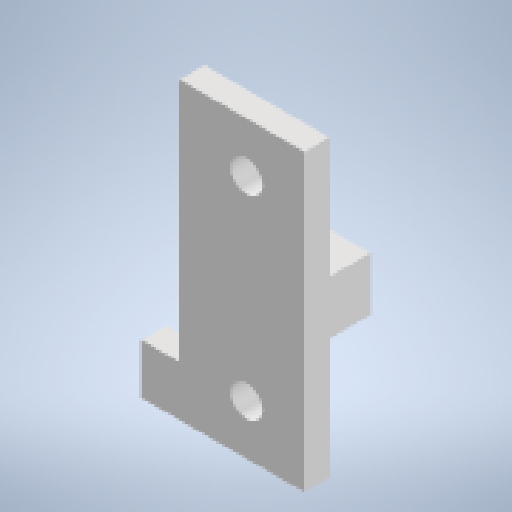
# Autodesk Inventor part: крышка
Saved by Autodesk Inventor 2024.2 (Build 282272000, 272)
## iProperties
Created: 2026-02-19
Part Number: крышка
Material: Типовые
Document SubType Name: Modeling
Designer: katya_notebook
Density: 1 g/cm^3
Appearance: По умолчанию
Author: katya_notebook
Autodesk Inventor part; units mm, degrees
ref_plane "YZ Plane" through (0, 0, 0) normal (1, 0, 0) x (0, 1, 0)
ref_plane "XZ Plane" through (0, 0, 0) normal (0, 1, 0) x (-1, 0, 0)
sketch "Эскиз1" plane through (0, 0, 0) normal (0, 0, 1) x (1, 0, 0)
  circle A0 centre (0.3813, 7.7585) radius 1.25 projected
  line L0 (-4.9754, 3.7665) -> (-4.9754, 11.75) projected
  line L1 (5, 3.7665) -> (-4.9754, 3.7665) projected
  line L2 (5, 11.75) -> (5, 3.7665) projected
  line L3 (-4.9754, 11.75) -> (5, 11.75) projected
  arc A1 (1.6313, -7.75) -> (-0.8686, -7.75) centre (0.3813, -7.762) ccw projected
  line L4 (-0.8686, -7.75) -> (1.6313, -7.75) projected
  line L5 (5, -11.75) -> (-8, -11.75) projected
  line L6 (5, -3.7735) -> (5, -11.75) projected
  line L7 (-5, -3.7735) -> (5, -3.7735) projected
  line L8 (-5, -7.75) -> (-5, -3.7735) projected
  line L9 (-8, -7.75) -> (-5, -7.75) projected
  line L10 (-8, -11.75) -> (-8, -7.75) projected
  line L11 (3.0114, -0.7535) -> (3.0052, -0.7535) projected
  line L12 (3.0114, -0.7535) -> (3.0114, -0.7535) projected
  arc A2 (3.5595, -1.3518) -> (3.0114, -0.7535) centre (3.0062, -1.3085) ccw projected
  arc A3 (3.5595, -1.3518) -> (3.709, -1.5135) centre (3.709, -1.3635) ccw projected
  line L13 (4.3002, -1.5135) -> (3.709, -1.5135) projected
  arc A4 (4.3002, -1.5135) -> (4.4502, -1.3635) centre (4.3002, -1.3635) ccw projected
  line L14 (4.4502, -1.2761) -> (4.4502, -1.3635) projected
  line L15 (4.4521, -1.2761) -> (4.4502, -1.2761) projected
  arc A5 (5, -0.7535) -> (4.4521, -1.2761) centre (5.0062, -1.3085) ccw projected
  line L16 (5, 0.7465) -> (5, -0.7535) projected
  arc A6 (4.4521, 1.2691) -> (5, 0.7465) centre (5.0062, 1.3015) ccw projected
  line L17 (4.4502, 1.2691) -> (4.4521, 1.2691) projected
  line L18 (4.4502, 1.3565) -> (4.4502, 1.2691) projected
  arc A7 (4.4502, 1.3565) -> (4.3002, 1.5065) centre (4.3002, 1.3565) ccw projected
  line L19 (3.709, 1.5065) -> (4.3002, 1.5065) projected
  arc A8 (3.709, 1.5065) -> (3.5595, 1.3448) centre (3.709, 1.3565) ccw projected
  arc A9 (3.0114, 0.7465) -> (3.5595, 1.3448) centre (3.0062, 1.3015) ccw projected
  line L20 (3.0114, 0.7465) -> (3.0114, 0.7465) projected
  line L21 (3.0052, 0.7465) -> (3.0114, 0.7465) projected
  line L22 (3.0052, 0.7465) -> (3.0052, 0.7465) projected
  arc A10 (2.4583, 1.2691) -> (3.0052, 0.7465) centre (3.0123, 1.3015) ccw projected
  line L23 (2.4564, 1.2691) -> (2.4583, 1.2691) projected
  line L24 (2.4564, 1.3565) -> (2.4564, 1.2691) projected
  arc A11 (2.4564, 1.3565) -> (2.3064, 1.5065) centre (2.3064, 1.3565) ccw projected
  line L25 (1.7152, 1.5065) -> (2.3064, 1.5065) projected
  arc A12 (1.7152, 1.5065) -> (1.5656, 1.3448) centre (1.7152, 1.3565) ccw projected
  arc A13 (1.0175, 0.7465) -> (1.5656, 1.3448) centre (1.0123, 1.3015) ccw projected
  line L26 (1.0175, 0.7465) -> (1.0175, 0.7465) projected
  line L27 (1.0114, 0.7465) -> (1.0175, 0.7465) projected
  line L28 (1.0114, 0.7465) -> (1.0114, 0.7465) projected
  arc A14 (0.4644, 1.2691) -> (1.0114, 0.7465) centre (1.0185, 1.3015) ccw projected
  line L29 (0.4625, 1.2691) -> (0.4644, 1.2691) projected
  line L30 (0.4625, 1.3565) -> (0.4625, 1.2691) projected
  arc A15 (0.4625, 1.3565) -> (0.3125, 1.5065) centre (0.3125, 1.3565) ccw projected
  line L31 (-0.2787, 1.5065) -> (0.3125, 1.5065) projected
  arc A16 (-0.2787, 1.5065) -> (-0.4282, 1.3448) centre (-0.2787, 1.3565) ccw projected
  arc A17 (-0.9763, 0.7465) -> (-0.4282, 1.3448) centre (-0.9815, 1.3015) ccw projected
  line L32 (-0.9763, 0.7465) -> (-0.9763, 0.7465) projected
  line L33 (-0.9825, 0.7465) -> (-0.9763, 0.7465) projected
  line L34 (-0.9825, 0.7465) -> (-0.9825, 0.7465) projected
  arc A18 (-1.5294, 1.2691) -> (-0.9825, 0.7465) centre (-0.9754, 1.3015) ccw projected
  line L35 (-1.5313, 1.2691) -> (-1.5294, 1.2691) projected
  line L36 (-1.5313, 1.3565) -> (-1.5313, 1.2691) projected
  arc A19 (-1.5313, 1.3565) -> (-1.6813, 1.5065) centre (-1.6813, 1.3565) ccw projected
  line L37 (-2.2725, 1.5065) -> (-1.6813, 1.5065) projected
  arc A20 (-2.2725, 1.5065) -> (-2.4221, 1.3448) centre (-2.2725, 1.3565) ccw projected
  arc A21 (-2.9754, 0.7465) -> (-2.4221, 1.3448) centre (-2.9754, 1.3015) ccw projected
  line L38 (-2.9754, 0.7465) -> (-2.9754, 2.2665) projected
  line L39 (5, 2.2665) -> (-2.9754, 2.2665) projected
  line L40 (5, 3.7665) -> (5, 2.2665) projected
  line L41 (-4.9754, 3.7665) -> (5, 3.7665) projected
  line L42 (-4.9754, -3.7735) -> (-4.9754, 3.7665) projected
  line L43 (5, -3.7735) -> (-4.9754, -3.7735) projected
  line L44 (5, -2.2735) -> (5, -3.7735) projected
  line L45 (-2.9754, -2.2735) -> (5, -2.2735) projected
  line L46 (-2.9754, -2.2735) -> (-2.9754, -0.7535) projected
  arc A22 (-2.4221, -1.3518) -> (-2.9754, -0.7535) centre (-2.9754, -1.3085) ccw projected
  arc A23 (-2.4221, -1.3518) -> (-2.2725, -1.5135) centre (-2.2725, -1.3635) ccw projected
  line L47 (-1.6813, -1.5135) -> (-2.2725, -1.5135) projected
  arc A24 (-1.6813, -1.5135) -> (-1.5313, -1.3635) centre (-1.6813, -1.3635) ccw projected
  line L48 (-1.5313, -1.2761) -> (-1.5313, -1.3635) projected
  line L49 (-1.5294, -1.2761) -> (-1.5313, -1.2761) projected
  arc A25 (-0.9825, -0.7535) -> (-1.5294, -1.2761) centre (-0.9754, -1.3085) ccw projected
  line L50 (-0.9825, -0.7535) -> (-0.9825, -0.7535) projected
  line L51 (-0.9763, -0.7535) -> (-0.9825, -0.7535) projected
  line L52 (-0.9763, -0.7535) -> (-0.9763, -0.7535) projected
  arc A26 (-0.4282, -1.3518) -> (-0.9763, -0.7535) centre (-0.9815, -1.3085) ccw projected
  arc A27 (-0.4282, -1.3518) -> (-0.2787, -1.5135) centre (-0.2787, -1.3635) ccw projected
  line L53 (0.3125, -1.5135) -> (-0.2787, -1.5135) projected
  arc A28 (0.3125, -1.5135) -> (0.4625, -1.3635) centre (0.3125, -1.3635) ccw projected
  line L54 (0.4625, -1.2761) -> (0.4625, -1.3635) projected
  line L55 (0.4644, -1.2761) -> (0.4625, -1.2761) projected
  arc A29 (1.0114, -0.7535) -> (0.4644, -1.2761) centre (1.0185, -1.3085) ccw projected
  line L56 (1.0114, -0.7535) -> (1.0114, -0.7535) projected
  line L57 (1.0175, -0.7535) -> (1.0114, -0.7535) projected
  line L58 (1.0175, -0.7535) -> (1.0175, -0.7535) projected
  arc A30 (1.5656, -1.3518) -> (1.0175, -0.7535) centre (1.0123, -1.3085) ccw projected
  arc A31 (1.5656, -1.3518) -> (1.7152, -1.5135) centre (1.7152, -1.3635) ccw projected
  line L59 (2.3064, -1.5135) -> (1.7152, -1.5135) projected
  arc A32 (2.3064, -1.5135) -> (2.4564, -1.3635) centre (2.3064, -1.3635) ccw projected
  line L60 (2.4564, -1.2761) -> (2.4564, -1.3635) projected
  line L61 (2.4583, -1.2761) -> (2.4564, -1.2761) projected
  arc A33 (3.0052, -0.7535) -> (2.4583, -1.2761) centre (3.0123, -1.3085) ccw projected
  line L62 (3.0052, -0.7535) -> (3.0052, -0.7535) projected
  circle A34 centre (0.3813, -7.762) radius 1.25
  line L63 (5, 2.2665) -> (5, -2.2735)
  point P0 (0, 0)
  point P1 (5, -0.7535)
  point P2 (-0.8686, -7.75)
  constraints: 2 end point, 1 coincident, 1 vertical, 3 other
extrude "Выдавливание1" add sketch "Эскиз1" along normal blind 2
sketch "Эскиз2" plane through (0, 0, 0) normal (0, 0, -1) x (-1, 0, 0)
  line L0 (-5, 2.2665) -> (-5, 0.7465) projected
  line L1 (-3.0114, -0.7535) -> (-3.0052, -0.7535) projected
  line L2 (-3.0114, -0.7535) -> (-3.0114, -0.7535) projected
  arc A0 (-3.0114, -0.7535) -> (-3.5595, -1.3518) centre (-3.0062, -1.3085) ccw projected
  arc A1 (-3.709, -1.5135) -> (-3.5595, -1.3518) centre (-3.709, -1.3635) ccw projected
  line L3 (-4.3002, -1.5135) -> (-3.709, -1.5135) projected
  arc A2 (-4.4502, -1.3635) -> (-4.3002, -1.5135) centre (-4.3002, -1.3635) ccw projected
  line L4 (-4.4502, -1.2761) -> (-4.4502, -1.3635) projected
  line L5 (-4.4521, -1.2761) -> (-4.4502, -1.2761) projected
  arc A3 (-4.4521, -1.2761) -> (-5, -0.7535) centre (-5.0062, -1.3085) ccw projected
  line L6 (-5, 0.7465) -> (-5, -0.7535) projected
  arc A4 (-5, 0.7465) -> (-4.4521, 1.2691) centre (-5.0062, 1.3015) ccw projected
  line L7 (-4.4502, 1.2691) -> (-4.4521, 1.2691) projected
  line L8 (-4.4502, 1.3565) -> (-4.4502, 1.2691) projected
  arc A5 (-4.3002, 1.5065) -> (-4.4502, 1.3565) centre (-4.3002, 1.3565) ccw projected
  line L9 (-3.709, 1.5065) -> (-4.3002, 1.5065) projected
  arc A6 (-3.5595, 1.3448) -> (-3.709, 1.5065) centre (-3.709, 1.3565) ccw projected
  arc A7 (-3.5595, 1.3448) -> (-3.0114, 0.7465) centre (-3.0062, 1.3015) ccw projected
  line L10 (-3.0114, 0.7465) -> (-3.0114, 0.7465) projected
  line L11 (-3.0052, 0.7465) -> (-3.0114, 0.7465) projected
  line L12 (-3.0052, 0.7465) -> (-3.0052, 0.7465) projected
  arc A8 (-3.0052, 0.7465) -> (-2.4583, 1.2691) centre (-3.0123, 1.3015) ccw projected
  line L13 (-2.4564, 1.2691) -> (-2.4583, 1.2691) projected
  line L14 (-2.4564, 1.3565) -> (-2.4564, 1.2691) projected
  arc A9 (-2.3064, 1.5065) -> (-2.4564, 1.3565) centre (-2.3064, 1.3565) ccw projected
  line L15 (-1.7152, 1.5065) -> (-2.3064, 1.5065) projected
  arc A10 (-1.5656, 1.3448) -> (-1.7152, 1.5065) centre (-1.7152, 1.3565) ccw projected
  arc A11 (-1.5656, 1.3448) -> (-1.0175, 0.7465) centre (-1.0123, 1.3015) ccw projected
  line L16 (-1.0175, 0.7465) -> (-1.0175, 0.7465) projected
  line L17 (-1.0114, 0.7465) -> (-1.0175, 0.7465) projected
  line L18 (-1.0114, 0.7465) -> (-1.0114, 0.7465) projected
  arc A12 (-1.0114, 0.7465) -> (-0.4644, 1.2691) centre (-1.0185, 1.3015) ccw projected
  line L19 (-0.4625, 1.2691) -> (-0.4644, 1.2691) projected
  line L20 (-0.4625, 1.3565) -> (-0.4625, 1.2691) projected
  arc A13 (-0.3125, 1.5065) -> (-0.4625, 1.3565) centre (-0.3125, 1.3565) ccw projected
  line L21 (0.2787, 1.5065) -> (-0.3125, 1.5065) projected
  arc A14 (0.4282, 1.3448) -> (0.2787, 1.5065) centre (0.2787, 1.3565) ccw projected
  arc A15 (0.4282, 1.3448) -> (0.9763, 0.7465) centre (0.9815, 1.3015) ccw projected
  line L22 (0.9763, 0.7465) -> (0.9763, 0.7465) projected
  line L23 (0.9825, 0.7465) -> (0.9763, 0.7465) projected
  line L24 (0.9825, 0.7465) -> (0.9825, 0.7465) projected
  arc A16 (0.9825, 0.7465) -> (1.5294, 1.2691) centre (0.9754, 1.3015) ccw projected
  line L25 (1.5313, 1.2691) -> (1.5294, 1.2691) projected
  line L26 (1.5313, 1.3565) -> (1.5313, 1.2691) projected
  arc A17 (1.6813, 1.5065) -> (1.5313, 1.3565) centre (1.6813, 1.3565) ccw projected
  line L27 (2.2725, 1.5065) -> (1.6813, 1.5065) projected
  arc A18 (2.4221, 1.3448) -> (2.2725, 1.5065) centre (2.2725, 1.3565) ccw projected
  arc A19 (2.4221, 1.3448) -> (2.9754, 0.7465) centre (2.9754, 1.3015) ccw projected
  line L28 (2.9754, 0.7465) -> (2.9754, 2.2665) projected
  line L29 (-5, 2.2665) -> (2.9754, 2.2665) projected
  line L30 (-5, 3.7665) -> (-5, 2.2665) projected
  line L31 (4.9754, 3.7665) -> (-5, 3.7665) projected
  line L32 (4.9754, -3.7735) -> (4.9754, 3.7665) projected
  line L33 (-5, -3.7735) -> (4.9754, -3.7735) projected
  line L34 (-5, -2.2735) -> (-5, -3.7735) projected
  line L35 (2.9754, -2.2735) -> (-5, -2.2735) projected
  line L36 (2.9754, -2.2735) -> (2.9754, -0.7535) projected
  arc A20 (2.9754, -0.7535) -> (2.4221, -1.3518) centre (2.9754, -1.3085) ccw projected
  arc A21 (2.2725, -1.5135) -> (2.4221, -1.3518) centre (2.2725, -1.3635) ccw projected
  line L37 (1.6813, -1.5135) -> (2.2725, -1.5135) projected
  arc A22 (1.5313, -1.3635) -> (1.6813, -1.5135) centre (1.6813, -1.3635) ccw projected
  line L38 (1.5313, -1.2761) -> (1.5313, -1.3635) projected
  line L39 (1.5294, -1.2761) -> (1.5313, -1.2761) projected
  arc A23 (1.5294, -1.2761) -> (0.9825, -0.7535) centre (0.9754, -1.3085) ccw projected
  line L40 (0.9825, -0.7535) -> (0.9825, -0.7535) projected
  line L41 (0.9763, -0.7535) -> (0.9825, -0.7535) projected
  line L42 (0.9763, -0.7535) -> (0.9763, -0.7535) projected
  arc A24 (0.9763, -0.7535) -> (0.4282, -1.3518) centre (0.9815, -1.3085) ccw projected
  arc A25 (0.2787, -1.5135) -> (0.4282, -1.3518) centre (0.2787, -1.3635) ccw projected
  line L43 (-0.3125, -1.5135) -> (0.2787, -1.5135) projected
  arc A26 (-0.4625, -1.3635) -> (-0.3125, -1.5135) centre (-0.3125, -1.3635) ccw projected
  line L44 (-0.4625, -1.2761) -> (-0.4625, -1.3635) projected
  line L45 (-0.4644, -1.2761) -> (-0.4625, -1.2761) projected
  arc A27 (-0.4644, -1.2761) -> (-1.0114, -0.7535) centre (-1.0185, -1.3085) ccw projected
  line L46 (-1.0114, -0.7535) -> (-1.0114, -0.7535) projected
  line L47 (-1.0175, -0.7535) -> (-1.0114, -0.7535) projected
  line L48 (-1.0175, -0.7535) -> (-1.0175, -0.7535) projected
  arc A28 (-1.0175, -0.7535) -> (-1.5656, -1.3518) centre (-1.0123, -1.3085) ccw projected
  arc A29 (-1.7152, -1.5135) -> (-1.5656, -1.3518) centre (-1.7152, -1.3635) ccw projected
  line L49 (-2.3064, -1.5135) -> (-1.7152, -1.5135) projected
  arc A30 (-2.4564, -1.3635) -> (-2.3064, -1.5135) centre (-2.3064, -1.3635) ccw projected
  line L50 (-2.4564, -1.2761) -> (-2.4564, -1.3635) projected
  line L51 (-2.4583, -1.2761) -> (-2.4564, -1.2761) projected
  arc A31 (-2.4583, -1.2761) -> (-3.0052, -0.7535) centre (-3.0123, -1.3085) ccw projected
  line L52 (-3.0052, -0.7535) -> (-3.0052, -0.7535) projected
  line L53 (-5, -11.75) -> (-5, 11.75) projected
  line L54 (-5, -2.1382) -> (-5, 2.1409)
  line L55 (-5, -2.1382) -> (2.6046, -2.1382)
  line L56 (2.6046, -2.1382) -> (2.6046, 2.1409)
  line L57 (-5, 2.1409) -> (2.6046, 2.1409)
  line L58 (-5, -11.75) -> (-5, 11.75) projected
  point P0 (0, 0)
  constraints: 8 end point, 3 perpendicular, 2 horizontal, 1 point on line, 4 other
ref_plane "РабПлоскость1" through (-4.9754, -3.7735, -3.25) normal (0, 0, 1) x (1, 0, 0)
extrude "Выдавливание2" add sketch "Эскиз2" along normal up to surface (3.25 mm away) contours L57 L56 A19 A18 L27 A17 L26 A16 L23 A15 A14 L21 A13 L20 A12 L17 A11 A10 L15 A9 L14 A8 L11 A7 A6 L9 A5 L8 A4 L0 | A4 L8 A5 L9 A6 A7 L11 A8 L14 A9 L15 A10 A11 L17 A12 L20 A13 L21 A14 A15 L23 A16 L26 A17 L27 A18 A19 L56 A20 A21 L37 A22 L38 A23 L41 A24 A25 L43 A26 L44 A27 L47 A28 A29 L49 A30 L50 A31 L1 A0 A1 L3 A2 L4 A3 L6 | A3 L4 A2 L3 A1 A0 L1 A31 L50 A30 L49 A29 A28 L47 A27 L44 A26 L43 A25 A24 L41 A23 L38 A22 L37 A21 A20 L56 L55 L53
